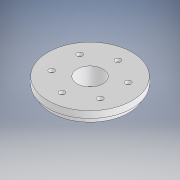
# Autodesk Inventor part: Cover
Saved by Autodesk Inventor 2017 SP1 (Build 210196100, 196)
## iProperties
Created: 2017-09-23
Part Number: Cover
Material: ABS Plastic
Document SubType Name: Modeling
Designer: Zach
Categories: <?xml version="1.0" encoding="UTF-16"?> <MemberInstance><Categories><FamilyTemplate><FamilyTemplateParameter ValueType="xs:double" Id="1" ObjectReferenceKey="da_z" ObjectType="kUserParameterObject"/><FamilyTemplateParameter ValueType="xs:double" Id="2" ObjectReferenceKey="da_b" ObjectType="kUserParameterObject"/><FamilyTemplateParameter ValueType="xs:double" Id="3" ObjectReferenceKey="da_beta" ObjectType="kUserParameterObject"/><FamilyTemplateParameter ValueType="xs:double" Id="4" ObjectReferenceKey="da_da" ObjectType="kUserParameterObject"/><FamilyTemplateParameter ValueType="xs:double" Id="5" ObjectReferenceKey="da_aw" ObjectType="kUserParameterObject"/><FamilyTemplateParameter ValueType="xs:string" Id="6" ObjectReferenceKey="EAIAABAAAACIAQAAAAAAAIAAAAAAAAAA" ObjectType="83910656" SubObjectId="SurfaceGeometry"/></FamilyTemplate><ParamToTemplateMap><ParamToTemplate CategoryParameter="//CategoryParameter[@InternalName='046C89C9-8512-4d59-83FE-43B91F4F132A']" TemplateParameter="1"/><ParamToTemplate CategoryParameter="//CategoryParameter[@InternalName='2552DF32-E462-4b46-AEBF-C6C7768E72AC']" TemplateParameter="2"/><ParamToTemplate CategoryParameter="//CategoryParameter[@InternalName='C9EE641D-15FC-4fae-A226-E94C4372FDD7']" TemplateParameter="3"/><ParamToTemplate><ParamToTemplate CategoryParameter="//CategoryParameter[@InternalName='00B6519A-459B-49c7-AD84-2E56D39A5744']" ConstantValue="-0.250000"/></ParamToTemplate><ParamToTemplate><ParamToTemplate CategoryParameter="//CategoryParameter[@InternalName='04B31F0E-C7A6-4894-AA32-9629BEFACF47']" ConstantValue="1.000000"/></ParamToTemplate><ParamToTemplate><ParamToTemplate CategoryParameter="//CategoryParameter[@InternalName='43CBEC2E-7847-49e7-A936-2F7889FCB2D9']" ConstantValue="0.250000"/></ParamToTemplate><ParamToTemplate><ParamToTemplate CategoryParameter="//CategoryParameter[@InternalName='B1EFC894-105D-4ebd-86BF-FA20ED196853']" ConstantValue="0.350000"/></ParamToTemplate><ParamToTemplate><ParamToTemplate CategoryParameter="//CategoryParameter[@InternalName='51175063-3D10-4879-93E8-6246FE8B403D']" ConstantValue="2060000000.000000"/></ParamToTemplate><ParamToTemplate><ParamToTemplate CategoryParameter="//CategoryParameter[@InternalName='A3A52E27-4454-46a9-B0BD-C932399B70AF']" ConstantValue="0.300000"/></ParamToTemplate><ParamToTemplate><ParamToTemplate CategoryParameter="//CategoryParameter[@InternalName='91B76062-C214-41d9-B1B9-14D2AB99603D']" ConstantValue="0.100000"/></ParamToTemplate><ParamToTemplate><ParamToTemplate CategoryParameter="//CategoryParameter[@InternalName='374E806E-8B8A-4dda-A9AA-1039D6500AD2']" ConstantValue="10.000000"/></ParamToTemplate><ParamToTemplate><ParamToTemplate CategoryParameter="//CategoryParameter[@InternalName='2D373A89-B862-43d6-8D0B-0CBF12AB9F6C']" ConstantValue="0.392699"/></ParamToTemplate><ParamToTemplate CategoryParameter="//CategoryParameter[@InternalName='37777632-D6A2-4fac-9D53-DB8ACD95C989']" TemplateParameter="4"/><ParamToTemplate CategoryParameter="//CategoryParameter[@InternalName='FD1017F1-B727-4f7e-9707-0F86F1FF9423']" TemplateParameter="5"/><ParamToTemplate><ParamToTemplate CategoryParameter="//CategoryParameter[@InternalName='9E1B4470-B2D3-4ff1-B813-535BB4CDF51A']" ConstantValue="3520000.000000"/></ParamToTemplate><ParamToTemplate><ParamToTemplate CategoryParameter="//CategoryParameter[@InternalName='F8452263-BFF6-458c-9FB1-07C4B99E95CD']" ConstantValue="11400000.000000"/></ParamToTemplate><ParamToTemplate><ParamToTemplate CategoryParameter="//CategoryParameter[@InternalName='3E3BB259-FD49-497f-8171-6EBC954A3479']" ConstantValue="2.000000"/></ParamToTemplate><ParamToTemplate CategoryParameter="//CategoryParameter[@InternalName='27C3BAF2-7550-4e4b-AE2C-0DB134B7D9B7']" TemplateParameter="6"/></ParamToTemplateMap><Category DisplayName="Gear" InternalName="DC85795E-93AB-48d5-8EEE-5A27447B64BD" Mnemonic="Gear"><CategoryParameter DisplayName="z" InternalName="046C89C9-8512-4d59-83FE-43B91F4F132A" Mnemonic="z"/><CategoryParameter DisplayName="b" InternalName="2552DF32-E462-4b46-AEBF-C6C7768E72AC" Mnemonic="b"/><CategoryParameter DisplayName="||b|" InternalName="C9EE641D-15FC-4fae-A226-E94C4372FDD7" Mnemonic="beta"/><CategoryParameter DisplayName="x" InternalName="00B6519A-459B-49c7-AD84-2E56D39A5744" Mnemonic="x"/><CategoryParameter DisplayName="a*" InternalName="04B31F0E-C7A6-4894-AA32-9629BEFACF47" Mnemonic="a"/><CategoryParameter DisplayName="c*" InternalName="43CBEC2E-7847-49e7-A936-2F7889FCB2D9" Mnemonic="c"/><CategoryParameter DisplayName="r|.f|*" InternalName="B1EFC894-105D-4ebd-86BF-FA20ED196853" Mnemonic="rf"/><CategoryParameter DisplayName="E" InternalName="51175063-3D10-4879-93E8-6246FE8B403D" Mnemonic="E"/><CategoryParameter DisplayName="||m|" InternalName="A3A52E27-4454-46a9-B0BD-C932399B70AF" Mnemonic="mi"/><Category DisplayName="SpurGear" InternalName="26C5A22E-A91E-4dfd-A3B3-23CCAFAE1764" Mnemonic="SpurGear"><CategoryParameter DisplayName="m" InternalName="91B76062-C214-41d9-B1B9-14D2AB99603D" Mnemonic="m"/><CategoryParameter DisplayName="P" InternalName="374E806E-8B8A-4dda-A9AA-1039D6500AD2" Mnemonic="PP"/><CategoryParameter DisplayName="||a|" InternalName="2D373A89-B862-43d6-8D0B-0CBF12AB9F6C" Mnemonic="alpha"/><CategoryParameter DisplayName="d|.a|" InternalName="37777632-D6A2-4fac-9D53-DB8ACD95C989" Mnemonic="da"/><CategoryParameter DisplayName="a|.w|" InternalName="FD1017F1-B727-4f7e-9707-0F86F1FF9423" Mnemonic="aw"/><CategoryParameter DisplayName="||s||.Flim|" InternalName="9E1B4470-B2D3-4ff1-B813-535BB4CDF51A" Mnemonic="sFlim"/><CategoryParameter DisplayName="||s||.Hlim|" InternalName="F8452263-BFF6-458c-9FB1-07C4B99E95CD" Mnemonic="sHlim"/><CategoryParameter DisplayName="type" InternalName="3E3BB259-FD49-497f-8171-6EBC954A3479" Mnemonic="type"/><CategoryParameter DisplayName="PitchDiameter" InternalName="27C3BAF2-7550-4e4b-AE2C-0DB134B7D9B7" Mnemonic="IDS_PITCHDIAM"/></Category></Category></Categories></MemberInstance>
Density: 1.06 g/cm^3
Appearance: CR White
CustomPartVersion: 1
Author: Zach
Autodesk Inventor part; units mm, degrees
sketch "Sketch1" plane through (0, 0, 0) normal (0, 0, 1) x (1, 0, 0)
  circle A0 centre (0, 0) radius 14.25
  dimension "d0" = 28.5
  constraints: 1 centre point
  measures "d0" diameter of A0
extrude "Extrusion1" add sketch "Sketch1" along normal blind 15
ref_plane "Work Plane2" through (0, 0, 7.5) normal (0, 0, 1) x (1, 0, 0)
sketch "Sketch2" plane through (0, 0, 0) normal (0, 0, -1) x (-1, 0, 0)
  circle A0 centre (0, 0) radius 14.25 projected
  circle A1 centre (0, 0) radius 13.5
  dimension "d3" = 27
  constraints: 1 centre point, 1 coincident
  measures "d3" diameter of A1
surface extrude "Pitch Diameter" sketch "Sketch2" against normal through all shown no curves A1
ref_plane "Work Plane8" through (0, 0, 0) normal (0.9932384, 0.1160929, 0) x (0, 0, 1)
ref_plane "Work Plane9" through (0, 0, 0) normal (1, 0, 0) x (0, 1, 0)
spur gear teeth "Spur Gear" teeth 27 pitch diameter 27 tip diameter 28.5 root diameter 24 face width 15 start plane through (0, 0, 0) normal (0, 0, -1) x (-1, 0, 0)
sketch "Sketch3" plane through (0, 0, 15) normal (0, 0, 1) x (1, 0, 0)
  circle A0 centre (0, 0) radius 11.5
  dimension "d49" = 23
  constraints: 1 centre point, 1 coincident
  measures "d49" diameter of A0
extrude "Extrusion2" cut sketch "Sketch3" against normal through all
sketch "Sketch4" plane through (0, 0, 15) normal (0, 0, 1) x (1, 0, 0)
  circle A0 centre (0, 0) radius 37.5
  circle A1 centre (0, 0) radius 11.5
  dimension "d52" = 75
  dimension "d53" = 23
  constraints: 2 centre point, 2 coincident
  measures "d52" diameter of A0
  measures "d53" diameter of A1
extrude "Extrusion3" add sketch "Sketch4" along normal blind 6
sketch "Sketch5" plane through (0, 0, 0) normal (0, 0, -1) x (-1, 0, 0)
  circle A0 centre (0, 0) radius 11.5 projected
  circle A1 centre (0, 0) radius 4.5
  dimension "d56" = 9
  constraints: 1 centre point, 1 coincident
  measures "d56" diameter of A1
extrude "Extrusion4" add sketch "Sketch5" against normal blind 13
sketch "Sketch6" plane through (0, 0, 21) normal (0, 0, 1) x (1, 0, 0)
  circle A0 centre (0, -25) radius 2.5
  circle A1 centre (21.6506, -12.5) radius 2.5
  circle A2 centre (21.6506, 12.5) radius 2.5
  circle A3 centre (0, 25) radius 2.5
  circle A4 centre (-21.6506, 12.5) radius 2.5
  circle A5 centre (-21.6506, -12.5) radius 2.5
  point P0 (0, 0)
  dimension "d59" = 5
  dimension "d60" = 25
  dimension "d63" = 360
  constraints: 6 centre point, 1 vertical alignment, 13 other
  measures "d59" diameter of A0
  measures "d60" distance of A0.centre point (0, 0)
extrude "Extrusion5" cut sketch "Sketch6" against normal through all
sketch "Sketch7" plane through (0, 0, 15) normal (0, 0, -1) x (-1, 0, 0)
  circle A0 centre (0, 25) radius 6.5
  circle A1 centre (21.6506, 12.5) radius 6.5
  circle A2 centre (21.6506, -12.5) radius 6.5
  circle A3 centre (0, -25) radius 6.5
  circle A4 centre (-21.6506, -12.5) radius 6.5
  circle A5 centre (-21.6506, 12.5) radius 6.5
  point P0 (0, 0)
  dimension "d67" = 13
  dimension "d68" = 25
  dimension "d71" = 360
  constraints: 6 centre point, 1 vertical alignment, 13 other
  measures "d67" diameter of A0
  measures "d68" distance of point (0, 0) A0.centre
extrude "Extrusion6" cut sketch "Sketch7" against normal blind 3
sketch "Sketch8" plane through (0, 0, 13) normal (0, 0, 1) x (1, 0, 0)
  circle A0 centre (0, 0) radius 4.5 projected
  circle A1 centre (0, 0) radius 11.5 projected
extrude "Extrusion7" cut sketch "Sketch8" against normal blind 8
sketch "Sketch9" plane through (0, 0, 15) normal (0, 0, -1) x (-1, 0, 0)
  circle A0 centre (0, 0) radius 34.5
  circle A1 centre (-21.6506, -12.5) radius 6.5 projected
  circle A2 centre (21.6506, -12.5) radius 6.5 projected
  circle A3 centre (0, 25) radius 6.5 projected
  circle A4 centre (21.6506, 12.5) radius 6.5 projected
  circle A5 centre (0, -25) radius 6.5 projected
  circle A6 centre (-21.6506, 12.5) radius 6.5 projected
  circle A7 centre (0, 0) radius 37.5 construction
  arc A8 (1.7392, 11.8733) -> (1.0459, 11.9543) centre (0, 0) ccw projected
  arc A9 (2.8816, 13.9556) -> (1.7392, 11.8733) centre (10.676, 8.3248) ccw projected
  arc A10 (3.6882, 13.7644) -> (2.8816, 13.9556) centre (0, 0) ccw projected
  arc A11 (3.7745, 11.3909) -> (3.6882, 13.7644) centre (-5.8043, 12.2307) ccw projected
  arc A12 (4.4305, 11.1522) -> (3.7745, 11.3909) centre (0, 0) ccw projected
  arc A13 (6.0223, 12.9149) -> (4.4305, 11.1522) centre (12.3081, 5.6383) ccw projected
  arc A14 (6.7631, 12.5429) -> (6.0223, 12.9149) centre (0, 0) ccw projected
  arc A15 (6.2997, 10.2134) -> (6.7631, 12.5429) centre (-2.8272, 13.2396) ccw projected
  arc A16 (6.8829, 9.8298) -> (6.2997, 10.2134) centre (0, 0) ccw projected
  arc A17 (8.8384, 11.1779) -> (6.8829, 9.8298) centre (13.2766, 2.6479) ccw projected
  arc A18 (9.4733, 10.6451) -> (8.8384, 11.1779) centre (0, 0) ccw projected
  arc A19 (8.4853, 8.4853) -> (9.4733, 10.6451) centre (0.3022, 13.5347) ccw projected
  arc A20 (8.9643, 7.9776) -> (8.4853, 8.4853) centre (0, 0) ccw projected
  arc A21 (11.1779, 8.8384) -> (8.9643, 7.9776) centre (13.5294, -0.4852) ccw projected
  arc A22 (11.6729, 8.1735) -> (11.1779, 8.8384) centre (0, 0) ccw projected
  arc A23 (10.2134, 6.2997) -> (11.6729, 8.1735) centre (3.4154, 13.1002) ccw projected
  arc A24 (10.5624, 5.6952) -> (10.2134, 6.2997) centre (0, 0) ccw projected
  arc A25 (12.9149, 6.0223) -> (10.5624, 5.6952) centre (13.0528, -3.5923) ccw projected
  arc A26 (13.2432, 5.2612) -> (12.9149, 6.0223) centre (0, 0) ccw projected
  arc A27 (11.3909, 3.7745) -> (13.2432, 5.2612) centre (6.3445, 11.9594) ccw projected
  arc A28 (11.5911, 3.1058) -> (11.3909, 3.7745) centre (0, 0) ccw projected
  arc A29 (13.9556, 2.8816) -> (11.5911, 3.1058) centre (11.8725, -6.5056) ccw projected
  arc A30 (14.0995, 2.0653) -> (13.9556, 2.8816) centre (0, 0) ccw projected
  arc A31 (11.9543, 1.0459) -> (14.0995, 2.0653) centre (8.9315, 10.1739) ccw projected
  arc A32 (11.9949, 0.349) -> (11.9543, 1.0459) centre (0, 0) ccw projected
  arc A33 (14.244, -0.4145) -> (11.9949, 0.349) centre (10.0522, -9.0682) ccw projected
  arc A34 (14.1958, -1.242) -> (14.244, -0.4145) centre (0, 0) ccw projected
  arc A35 (11.8733, -1.7392) -> (14.1958, -1.242) centre (11.037, 7.8399) ccw projected
  arc A36 (11.7521, -2.4266) -> (11.8733, -1.7392) centre (0, 0) ccw projected
  arc A37 (13.7644, -3.6882) -> (11.7521, -2.4266) centre (7.69, -11.142) ccw projected
  arc A38 (13.5267, -4.4823) -> (13.7644, -3.6882) centre (0, 0) ccw projected
  arc A39 (11.1522, -4.4305) -> (13.5267, -4.4823) centre (12.5475, 5.0833) ccw projected
  arc A40 (10.8757, -5.0714) -> (11.1522, -4.4305) centre (0, 0) ccw projected
  arc A41 (12.5429, -6.7631) -> (10.8757, -5.0714) centre (4.9132, -12.6151) ccw projected
  arc A42 (12.1284, -7.4809) -> (12.5429, -6.7631) centre (0, 0) ccw projected
  arc A43 (9.8298, -6.8829) -> (12.1284, -7.4809) centre (13.3816, 2.0526) ccw projected
  arc A44 (9.413, -7.4428) -> (9.8298, -6.8829) centre (0, 0) ccw projected
  arc A45 (10.6451, -9.4733) -> (9.413, -7.4428) centre (1.8715, -13.4081) ccw projected
  arc A46 (10.0763, -10.0763) -> (10.6451, -9.4733) centre (0, 0) ccw projected
  arc A47 (7.9776, -8.9643) -> (10.0763, -10.0763) centre (13.4942, -1.0887) ccw projected
  arc A48 (7.4428, -9.413) -> (7.9776, -8.9643) centre (0, 0) ccw projected
  arc A49 (8.1735, -11.6729) -> (7.4428, -9.413) centre (-1.2711, -13.4783) ccw projected
  arc A50 (7.4809, -12.1284) -> (8.1735, -11.6729) centre (0, 0) ccw projected
  arc A51 (5.6952, -10.5624) -> (7.4809, -12.1284) centre (12.8794, -4.1713) ccw projected
  arc A52 (5.0714, -10.8757) -> (5.6952, -10.5624) centre (0, 0) ccw projected
  arc A53 (5.2612, -13.2432) -> (5.0714, -10.8757) centre (-4.3451, -12.8218) ccw projected
  arc A54 (4.4823, -13.5267) -> (5.2612, -13.2432) centre (0, 0) ccw projected
  arc A55 (3.1058, -11.5911) -> (4.4823, -13.5267) centre (11.5703, -7.0291) ccw projected
  arc A56 (2.4266, -11.7521) -> (3.1058, -11.5911) centre (0, 0) ccw projected
  arc A57 (2.0653, -14.0995) -> (2.4266, -11.7521) centre (-7.1849, -11.4742) ccw projected
  arc A58 (1.242, -14.1958) -> (2.0653, -14.0995) centre (0, 0) ccw projected
  arc A59 (0.349, -11.9949) -> (1.242, -14.1958) centre (9.6374, -9.5079) ccw projected
  arc A60 (-0.349, -11.9949) -> (0.349, -11.9949) centre (0, 0) ccw projected
  arc A61 (-1.242, -14.1958) -> (-0.349, -11.9949) centre (-9.6374, -9.5079) ccw projected
  arc A62 (-2.0653, -14.0995) -> (-1.242, -14.1958) centre (0, 0) ccw projected
  arc A63 (-2.4266, -11.7521) -> (-2.0653, -14.0995) centre (7.1849, -11.4742) ccw projected
  arc A64 (-3.1058, -11.5911) -> (-2.4266, -11.7521) centre (0, 0) ccw projected
  arc A65 (-4.4823, -13.5267) -> (-3.1058, -11.5911) centre (-11.5703, -7.0291) ccw projected
  arc A66 (-5.2612, -13.2432) -> (-4.4823, -13.5267) centre (0, 0) ccw projected
  arc A67 (-5.0714, -10.8757) -> (-5.2612, -13.2432) centre (4.3451, -12.8218) ccw projected
  arc A68 (-5.6952, -10.5624) -> (-5.0714, -10.8757) centre (0, 0) ccw projected
  arc A69 (-7.4809, -12.1284) -> (-5.6952, -10.5624) centre (-12.8794, -4.1713) ccw projected
  arc A70 (-8.1735, -11.6729) -> (-7.4809, -12.1284) centre (0, 0) ccw projected
  arc A71 (-7.4428, -9.413) -> (-8.1735, -11.6729) centre (1.2711, -13.4783) ccw projected
  arc A72 (-7.9776, -8.9643) -> (-7.4428, -9.413) centre (0, 0) ccw projected
  arc A73 (-10.0763, -10.0763) -> (-7.9776, -8.9643) centre (-13.4942, -1.0887) ccw projected
  arc A74 (-10.6451, -9.4733) -> (-10.0763, -10.0763) centre (0, 0) ccw projected
  arc A75 (-9.413, -7.4428) -> (-10.6451, -9.4733) centre (-1.8715, -13.4081) ccw projected
  arc A76 (-9.8298, -6.8829) -> (-9.413, -7.4428) centre (0, 0) ccw projected
  arc A77 (-12.1284, -7.4809) -> (-9.8298, -6.8829) centre (-13.3816, 2.0526) ccw projected
  arc A78 (-12.5429, -6.7631) -> (-12.1284, -7.4809) centre (0, 0) ccw projected
  arc A79 (-10.8757, -5.0714) -> (-12.5429, -6.7631) centre (-4.9132, -12.6151) ccw projected
  arc A80 (-11.1522, -4.4305) -> (-10.8757, -5.0714) centre (0, 0) ccw projected
  arc A81 (-13.5267, -4.4823) -> (-11.1522, -4.4305) centre (-12.5475, 5.0833) ccw projected
  arc A82 (-13.7644, -3.6882) -> (-13.5267, -4.4823) centre (0, 0) ccw projected
  arc A83 (-11.7521, -2.4266) -> (-13.7644, -3.6882) centre (-7.69, -11.142) ccw projected
  arc A84 (-11.8733, -1.7392) -> (-11.7521, -2.4266) centre (0, 0) ccw projected
  arc A85 (-14.1958, -1.242) -> (-11.8733, -1.7392) centre (-11.037, 7.8399) ccw projected
  arc A86 (-14.244, -0.4145) -> (-14.1958, -1.242) centre (0, 0) ccw projected
  arc A87 (-11.9949, 0.349) -> (-14.244, -0.4145) centre (-10.0522, -9.0682) ccw projected
  arc A88 (-11.9543, 1.0459) -> (-11.9949, 0.349) centre (0, 0) ccw projected
  arc A89 (-14.0995, 2.0653) -> (-11.9543, 1.0459) centre (-8.9315, 10.1739) ccw projected
  arc A90 (-13.9556, 2.8816) -> (-14.0995, 2.0653) centre (0, 0) ccw projected
  arc A91 (-11.5911, 3.1058) -> (-13.9556, 2.8816) centre (-11.8725, -6.5056) ccw projected
  arc A92 (-11.3909, 3.7745) -> (-11.5911, 3.1058) centre (0, 0) ccw projected
  arc A93 (-13.2432, 5.2612) -> (-11.3909, 3.7745) centre (-6.3445, 11.9594) ccw projected
  arc A94 (-12.9149, 6.0223) -> (-13.2432, 5.2612) centre (0, 0) ccw projected
  arc A95 (-10.5624, 5.6952) -> (-12.9149, 6.0223) centre (-13.0528, -3.5923) ccw projected
  arc A96 (-10.2134, 6.2997) -> (-10.5624, 5.6952) centre (0, 0) ccw projected
  arc A97 (-11.6729, 8.1735) -> (-10.2134, 6.2997) centre (-3.4154, 13.1002) ccw projected
  arc A98 (-11.1779, 8.8384) -> (-11.6729, 8.1735) centre (0, 0) ccw projected
  arc A99 (-8.9643, 7.9776) -> (-11.1779, 8.8384) centre (-13.5294, -0.4852) ccw projected
  arc A100 (-8.4853, 8.4853) -> (-8.9643, 7.9776) centre (0, 0) ccw projected
  arc A101 (-9.4733, 10.6451) -> (-8.4853, 8.4853) centre (-0.3022, 13.5347) ccw projected
  arc A102 (-8.8384, 11.1779) -> (-9.4733, 10.6451) centre (0, 0) ccw projected
  arc A103 (-6.8829, 9.8298) -> (-8.8384, 11.1779) centre (-13.2766, 2.6479) ccw projected
  arc A104 (-6.2997, 10.2134) -> (-6.8829, 9.8298) centre (0, 0) ccw projected
  arc A105 (-6.7631, 12.5429) -> (-6.2997, 10.2134) centre (2.8272, 13.2396) ccw projected
  arc A106 (-6.0223, 12.9149) -> (-6.7631, 12.5429) centre (0, 0) ccw projected
  arc A107 (-4.4305, 11.1522) -> (-6.0223, 12.9149) centre (-12.3081, 5.6383) ccw projected
  arc A108 (-3.7745, 11.3909) -> (-4.4305, 11.1522) centre (0, 0) ccw projected
  arc A109 (-3.6882, 13.7644) -> (-3.7745, 11.3909) centre (5.8043, 12.2307) ccw projected
  arc A110 (-2.8816, 13.9556) -> (-3.6882, 13.7644) centre (0, 0) ccw projected
  arc A111 (-1.7392, 11.8733) -> (-2.8816, 13.9556) centre (-10.676, 8.3248) ccw projected
  arc A112 (-1.0459, 11.9543) -> (-1.7392, 11.8733) centre (0, 0) ccw projected
  arc A113 (-0.4145, 14.244) -> (-1.0459, 11.9543) centre (8.4684, 10.5625) ccw projected
  arc A114 (0.4145, 14.244) -> (-0.4145, 14.244) centre (0, 0) ccw projected
  arc A115 (1.0459, 11.9543) -> (0.4145, 14.244) centre (-8.4684, 10.5625) ccw projected
  dimension "d77" = 69
  constraints: 1 centre point, 1 coincident
  measures "d77" diameter of A0
extrude "Extrusion8" add sketch "Sketch9" along normal blind 5
sketch "Sketch10" plane through (0, 0, 10) normal (0, 0, -1) x (-1, 0, 0)
  circle A0 centre (0, 0) radius 17.5
  circle A1 centre (0, 0) radius 4.5 projected
  arc A2 (3.7745, 11.3909) -> (3.6882, 13.7644) centre (-5.8043, 12.2307) ccw projected
  arc A3 (3.6882, 13.7644) -> (2.8816, 13.9556) centre (0, 0) ccw projected
  arc A4 (2.8816, 13.9556) -> (1.7392, 11.8733) centre (10.676, 8.3248) ccw projected
  arc A5 (1.7392, 11.8733) -> (1.0459, 11.9543) centre (0, 0) ccw projected
  arc A6 (1.0459, 11.9543) -> (0.4145, 14.244) centre (-8.4684, 10.5625) ccw projected
  arc A7 (0.4145, 14.244) -> (-0.4145, 14.244) centre (0, 0) ccw projected
  arc A8 (-0.4145, 14.244) -> (-1.0459, 11.9543) centre (8.4684, 10.5625) ccw projected
  arc A9 (-1.0459, 11.9543) -> (-1.7392, 11.8733) centre (0, 0) ccw projected
  arc A10 (-1.7392, 11.8733) -> (-2.8816, 13.9556) centre (-10.676, 8.3248) ccw projected
  arc A11 (-2.8816, 13.9556) -> (-3.6882, 13.7644) centre (0, 0) ccw projected
  arc A12 (-3.6882, 13.7644) -> (-3.7745, 11.3909) centre (5.8043, 12.2307) ccw projected
  arc A13 (-3.7745, 11.3909) -> (-4.4305, 11.1522) centre (0, 0) ccw projected
  arc A14 (-4.4305, 11.1522) -> (-6.0223, 12.9149) centre (-12.3081, 5.6383) ccw projected
  arc A15 (-6.0223, 12.9149) -> (-6.7631, 12.5429) centre (0, 0) ccw projected
  arc A16 (-6.7631, 12.5429) -> (-6.2997, 10.2134) centre (2.8272, 13.2396) ccw projected
  arc A17 (-6.2997, 10.2134) -> (-6.8829, 9.8298) centre (0, 0) ccw projected
  arc A18 (-6.8829, 9.8298) -> (-8.8384, 11.1779) centre (-13.2766, 2.6479) ccw projected
  arc A19 (-8.8384, 11.1779) -> (-9.4733, 10.6451) centre (0, 0) ccw projected
  arc A20 (-9.4733, 10.6451) -> (-8.4853, 8.4853) centre (-0.3022, 13.5347) ccw projected
  arc A21 (-8.4853, 8.4853) -> (-8.9643, 7.9776) centre (0, 0) ccw projected
  arc A22 (-8.9643, 7.9776) -> (-11.1779, 8.8384) centre (-13.5294, -0.4852) ccw projected
  arc A23 (-11.1779, 8.8384) -> (-11.6729, 8.1735) centre (0, 0) ccw projected
  arc A24 (-11.6729, 8.1735) -> (-10.2134, 6.2997) centre (-3.4154, 13.1002) ccw projected
  arc A25 (-10.2134, 6.2997) -> (-10.5624, 5.6952) centre (0, 0) ccw projected
  arc A26 (-10.5624, 5.6952) -> (-12.9149, 6.0223) centre (-13.0528, -3.5923) ccw projected
  arc A27 (-12.9149, 6.0223) -> (-13.2432, 5.2612) centre (0, 0) ccw projected
  arc A28 (-13.2432, 5.2612) -> (-11.3909, 3.7745) centre (-6.3445, 11.9594) ccw projected
  arc A29 (-11.3909, 3.7745) -> (-11.5911, 3.1058) centre (0, 0) ccw projected
  arc A30 (-11.5911, 3.1058) -> (-13.9556, 2.8816) centre (-11.8725, -6.5056) ccw projected
  arc A31 (-13.9556, 2.8816) -> (-14.0995, 2.0653) centre (0, 0) ccw projected
  arc A32 (-14.0995, 2.0653) -> (-11.9543, 1.0459) centre (-8.9315, 10.1739) ccw projected
  arc A33 (-11.9543, 1.0459) -> (-11.9949, 0.349) centre (0, 0) ccw projected
  arc A34 (-11.9949, 0.349) -> (-14.244, -0.4145) centre (-10.0522, -9.0682) ccw projected
  arc A35 (-14.244, -0.4145) -> (-14.1958, -1.242) centre (0, 0) ccw projected
  arc A36 (-14.1958, -1.242) -> (-11.8733, -1.7392) centre (-11.037, 7.8399) ccw projected
  arc A37 (-11.8733, -1.7392) -> (-11.7521, -2.4266) centre (0, 0) ccw projected
  arc A38 (-11.7521, -2.4266) -> (-13.7644, -3.6882) centre (-7.69, -11.142) ccw projected
  arc A39 (-13.7644, -3.6882) -> (-13.5267, -4.4823) centre (0, 0) ccw projected
  arc A40 (-13.5267, -4.4823) -> (-11.1522, -4.4305) centre (-12.5475, 5.0833) ccw projected
  arc A41 (-11.1522, -4.4305) -> (-10.8757, -5.0714) centre (0, 0) ccw projected
  arc A42 (-10.8757, -5.0714) -> (-12.5429, -6.7631) centre (-4.9132, -12.6151) ccw projected
  arc A43 (-12.5429, -6.7631) -> (-12.1284, -7.4809) centre (0, 0) ccw projected
  arc A44 (-12.1284, -7.4809) -> (-9.8298, -6.8829) centre (-13.3816, 2.0526) ccw projected
  arc A45 (-9.8298, -6.8829) -> (-9.413, -7.4428) centre (0, 0) ccw projected
  arc A46 (-9.413, -7.4428) -> (-10.6451, -9.4733) centre (-1.8715, -13.4081) ccw projected
  arc A47 (-10.6451, -9.4733) -> (-10.0763, -10.0763) centre (0, 0) ccw projected
  arc A48 (-10.0763, -10.0763) -> (-7.9776, -8.9643) centre (-13.4942, -1.0887) ccw projected
  arc A49 (-7.9776, -8.9643) -> (-7.4428, -9.413) centre (0, 0) ccw projected
  arc A50 (-7.4428, -9.413) -> (-8.1735, -11.6729) centre (1.2711, -13.4783) ccw projected
  arc A51 (-8.1735, -11.6729) -> (-7.4809, -12.1284) centre (0, 0) ccw projected
  arc A52 (-7.4809, -12.1284) -> (-5.6952, -10.5624) centre (-12.8794, -4.1713) ccw projected
  arc A53 (-5.6952, -10.5624) -> (-5.0714, -10.8757) centre (0, 0) ccw projected
  arc A54 (-5.0714, -10.8757) -> (-5.2612, -13.2432) centre (4.3451, -12.8218) ccw projected
  arc A55 (-5.2612, -13.2432) -> (-4.4823, -13.5267) centre (0, 0) ccw projected
  arc A56 (-4.4823, -13.5267) -> (-3.1058, -11.5911) centre (-11.5703, -7.0291) ccw projected
  arc A57 (-3.1058, -11.5911) -> (-2.4266, -11.7521) centre (0, 0) ccw projected
  arc A58 (-2.4266, -11.7521) -> (-2.0653, -14.0995) centre (7.1849, -11.4742) ccw projected
  arc A59 (-2.0653, -14.0995) -> (-1.242, -14.1958) centre (0, 0) ccw projected
  arc A60 (-1.242, -14.1958) -> (-0.349, -11.9949) centre (-9.6374, -9.5079) ccw projected
  arc A61 (-0.349, -11.9949) -> (0.349, -11.9949) centre (0, 0) ccw projected
  arc A62 (0.349, -11.9949) -> (1.242, -14.1958) centre (9.6374, -9.5079) ccw projected
  arc A63 (1.242, -14.1958) -> (2.0653, -14.0995) centre (0, 0) ccw projected
  arc A64 (2.0653, -14.0995) -> (2.4266, -11.7521) centre (-7.1849, -11.4742) ccw projected
  arc A65 (2.4266, -11.7521) -> (3.1058, -11.5911) centre (0, 0) ccw projected
  arc A66 (3.1058, -11.5911) -> (4.4823, -13.5267) centre (11.5703, -7.0291) ccw projected
  arc A67 (4.4823, -13.5267) -> (5.2612, -13.2432) centre (0, 0) ccw projected
  arc A68 (5.2612, -13.2432) -> (5.0714, -10.8757) centre (-4.3451, -12.8218) ccw projected
  arc A69 (5.0714, -10.8757) -> (5.6952, -10.5624) centre (0, 0) ccw projected
  arc A70 (5.6952, -10.5624) -> (7.4809, -12.1284) centre (12.8794, -4.1713) ccw projected
  arc A71 (7.4809, -12.1284) -> (8.1735, -11.6729) centre (0, 0) ccw projected
  arc A72 (8.1735, -11.6729) -> (7.4428, -9.413) centre (-1.2711, -13.4783) ccw projected
  arc A73 (7.4428, -9.413) -> (7.9776, -8.9643) centre (0, 0) ccw projected
  arc A74 (7.9776, -8.9643) -> (10.0763, -10.0763) centre (13.4942, -1.0887) ccw projected
  arc A75 (10.0763, -10.0763) -> (10.6451, -9.4733) centre (0, 0) ccw projected
  arc A76 (10.6451, -9.4733) -> (9.413, -7.4428) centre (1.8715, -13.4081) ccw projected
  arc A77 (9.413, -7.4428) -> (9.8298, -6.8829) centre (0, 0) ccw projected
  arc A78 (9.8298, -6.8829) -> (12.1284, -7.4809) centre (13.3816, 2.0526) ccw projected
  arc A79 (12.1284, -7.4809) -> (12.5429, -6.7631) centre (0, 0) ccw projected
  arc A80 (12.5429, -6.7631) -> (10.8757, -5.0714) centre (4.9132, -12.6151) ccw projected
  arc A81 (10.8757, -5.0714) -> (11.1522, -4.4305) centre (0, 0) ccw projected
  arc A82 (11.1522, -4.4305) -> (13.5267, -4.4823) centre (12.5475, 5.0833) ccw projected
  arc A83 (13.5267, -4.4823) -> (13.7644, -3.6882) centre (0, 0) ccw projected
  arc A84 (13.7644, -3.6882) -> (11.7521, -2.4266) centre (7.69, -11.142) ccw projected
  arc A85 (11.7521, -2.4266) -> (11.8733, -1.7392) centre (0, 0) ccw projected
  arc A86 (11.8733, -1.7392) -> (14.1958, -1.242) centre (11.037, 7.8399) ccw projected
  arc A87 (14.1958, -1.242) -> (14.244, -0.4145) centre (0, 0) ccw projected
  arc A88 (14.244, -0.4145) -> (11.9949, 0.349) centre (10.0522, -9.0682) ccw projected
  arc A89 (11.9949, 0.349) -> (11.9543, 1.0459) centre (0, 0) ccw projected
  arc A90 (11.9543, 1.0459) -> (14.0995, 2.0653) centre (8.9315, 10.1739) ccw projected
  arc A91 (14.0995, 2.0653) -> (13.9556, 2.8816) centre (0, 0) ccw projected
  arc A92 (13.9556, 2.8816) -> (11.5911, 3.1058) centre (11.8725, -6.5056) ccw projected
  arc A93 (11.5911, 3.1058) -> (11.3909, 3.7745) centre (0, 0) ccw projected
  arc A94 (11.3909, 3.7745) -> (13.2432, 5.2612) centre (6.3445, 11.9594) ccw projected
  arc A95 (13.2432, 5.2612) -> (12.9149, 6.0223) centre (0, 0) ccw projected
  arc A96 (12.9149, 6.0223) -> (10.5624, 5.6952) centre (13.0528, -3.5923) ccw projected
  arc A97 (10.5624, 5.6952) -> (10.2134, 6.2997) centre (0, 0) ccw projected
  arc A98 (10.2134, 6.2997) -> (11.6729, 8.1735) centre (3.4154, 13.1002) ccw projected
  arc A99 (11.6729, 8.1735) -> (11.1779, 8.8384) centre (0, 0) ccw projected
  arc A100 (11.1779, 8.8384) -> (8.9643, 7.9776) centre (13.5294, -0.4852) ccw projected
  arc A101 (8.9643, 7.9776) -> (8.4853, 8.4853) centre (0, 0) ccw projected
  arc A102 (8.4853, 8.4853) -> (9.4733, 10.6451) centre (0.3022, 13.5347) ccw projected
  arc A103 (9.4733, 10.6451) -> (8.8384, 11.1779) centre (0, 0) ccw projected
  arc A104 (8.8384, 11.1779) -> (6.8829, 9.8298) centre (13.2766, 2.6479) ccw projected
  arc A105 (6.8829, 9.8298) -> (6.2997, 10.2134) centre (0, 0) ccw projected
  arc A106 (6.2997, 10.2134) -> (6.7631, 12.5429) centre (-2.8272, 13.2396) ccw projected
  arc A107 (6.7631, 12.5429) -> (6.0223, 12.9149) centre (0, 0) ccw projected
  arc A108 (6.0223, 12.9149) -> (4.4305, 11.1522) centre (12.3081, 5.6383) ccw projected
  arc A109 (4.4305, 11.1522) -> (3.7745, 11.3909) centre (0, 0) ccw projected
  dimension "d80" = 35
  constraints: 1 centre point, 1 coincident
  measures "d80" diameter of A0
extrude "Extrusion9" add sketch "Sketch10" along normal blind 5 contours A0
equation "\"d0\" = da_da"
equation "\"d1\" = da_b"
equation "\"d3\" = da_dw"
equation "\"da_da\" = 28.5"
equation "\"da_b\" = 15"
equation "\"da_dw\" = 27"
body "Solid1"
body "Srf1"
